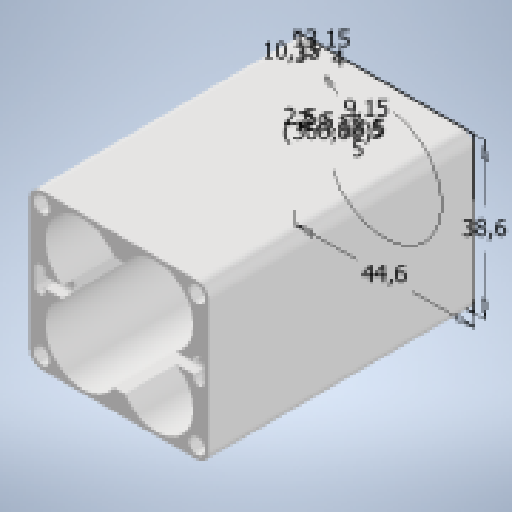
# Autodesk Inventor part: akkum
Saved by Autodesk Inventor 2025 (Build 290162000, 162)
## iProperties
Created: 2026-06-25
Part Number: akkum
Material: Типовые
Document SubType Name: Modeling
Designer: garin
Density: 1 g/cm^3
Appearance: По умолчанию
Author: garin
Autodesk Inventor part; units mm, degrees
ref_plane "YZ Plane" through (0, 0, 0) normal (1, 0, 0) x (0, 1, 0)
ref_plane "XZ Plane" through (0, 0, 0) normal (0, 1, 0) x (-1, 0, 0)
ref_plane "XY Plane" through (0, 0, 0) normal (0, 0, 1) x (1, 0, 0)
sketch "Эскиз1" plane through (0, 0, 0) normal (0, 0, 1) x (1, 0, 0)
  circle A0 centre (-9.15, 9.15) radius 9.25
  line L0 (0, 0) -> (-9.15, 0) construction
  line L1 (-9.15, 0) -> (-9.15, 9.15) construction
  line L2 (-9.15, 9.15) -> (0, 9.15) construction
  line L3 (0, 9.15) -> (0, 0) construction
  circle A1 centre (9.15, 9.15) radius 9.25
  circle A2 centre (-9.15, -9.15) radius 9.25
  circle A3 centre (9.15, -9.15) radius 9.25
  line L4 (0, 10.5065) -> (-0.6478, 10.5065) construction
  line L5 (-0.6478, 10.5065) -> (-0.6478, 5.5065) construction
  line L6 (-0.6478, 5.5065) -> (0, 5.5065) construction
  line L7 (0, 5.5065) -> (0, 10.5065) construction
  line L8 (-0.6478, 5.5065) -> (0.6478, 5.5065)
  line L9 (-0.6478, -5.5065) -> (0.6478, -5.5065)
  line L10 (-9.15, 0) -> (-4.15, 0) construction
  line L11 (-4.15, 0) -> (-4.15, 1.3678) construction
  line L12 (-4.15, 1.3678) -> (-9.15, 1.3678) construction
  line L13 (-9.15, 1.3678) -> (-9.15, 0) construction
  line L14 (-4.15, 1.3678) -> (-4.15, -1.3678)
  line L15 (4.15, 1.3678) -> (4.15, -1.3678)
  line L16 (-9.15, 9.15) -> (-22.3, 9.15) construction
  line L17 (-22.3, 9.15) -> (-22.3, 19.3) construction
  line L18 (-22.3, 19.3) -> (-9.15, 19.3) construction
  line L19 (-9.15, 19.3) -> (-9.15, 9.15) construction
  line L20 (-22.3, 19.3) -> (22.3, 19.3)
  line L21 (22.3, 19.3) -> (22.3, -19.3)
  line L22 (22.3, -19.3) -> (-22.3, -19.3)
  line L23 (-22.3, -19.3) -> (-22.3, 19.3)
  line L24 (-14.15, 1.3678) -> (-14.15, -1.3678)
  line L25 (14.15, 1.3678) -> (14.15, -1.3678)
  line L26 (-22.3, 19.3) -> (-19.3, 19.3) construction
  line L27 (-19.3, 19.3) -> (-19.3, 16.3) construction
  line L28 (-19.3, 16.3) -> (-22.3, 16.3) construction
  line L29 (-22.3, 16.3) -> (-22.3, 19.3) construction
  circle A4 centre (-19.3, 16.3) radius 2
  circle A5 centre (19.3, 16.3) radius 2
  circle A6 centre (-19.3, -16.3) radius 2
  circle A7 centre (19.3, -16.3) radius 2
  line L30 (-22.3, 0) -> (-19.8, 0) construction
  line L31 (-19.8, 0) -> (-19.8, 2) construction
  circle A8 centre (-19.8, 2) radius 1.25
  circle A9 centre (-19.8, -2) radius 1.25
  circle A10 centre (19.8, 2) radius 1.25
  circle A11 centre (19.8, -2) radius 1.25
  line L32 (-9.15, -9.15) -> (-22.3, -9.15) construction
  line L33 (-19.8, 2) -> (-21.05, 2) construction
  line L34 (-19.8, -2) -> (-21.05, -2) construction
  line L35 (-21.05, 2) -> (-21.05, -2)
  line L36 (-18.55, 2) -> (-18.55, -2)
  line L37 (21.05, 2) -> (21.05, -2)
  line L38 (18.55, 2) -> (18.55, -2)
  line L39 (14.15, 1.3678) -> (18.55, 1.3678)
  line L40 (14.15, -1.3678) -> (18.55, -1.3678)
  line L41 (-14.15, 1.3678) -> (-18.55, 1.3678)
  line L42 (-14.15, -1.3678) -> (-18.55, -1.3678)
  line L43 (-1.3678, -14.15) -> (1.3678, -14.15)
  line L44 (14.15, -1.3678) -> (14.15, 1.3678)
  line L45 (1.3678, 14.15) -> (-1.3678, 14.15)
  point P0 (14.15, 1.3678)
  point P1 (14.15, -1.3678)
  point P2 (-14.15, -1.3678)
  point P3 (-14.15, 1.3678)
  point P4 (4.15, -1.3678)
  point P5 (4.15, 1.3678)
  point P6 (-0.6478, -5.5065)
  point P7 (0.6478, -5.5065)
  point P8 (-18.55, -1.3678)
  point P9 (10.5065, 0)
  point P10 (0, -10.5065)
  point P11 (0, -7.7935)
  point P12 (-7.7935, 0)
  point P13 (-10.5065, 0)
  point P14 (7.7935, 0)
  point P15 (0, 7.7935)
  point P16 (0, 10.5065)
  dimension "d22" = 2.5
  dimension "d0" = 18.5
  dimension "d1" = 9.15
  dimension "d2" = 9.15
  dimension "d3" = 5
  dimension "d4" = 5
  dimension "d5" = 13.15
  dimension "d6" = 10.15
  dimension "d7" = 44.6
  dimension "d8" = 38.6
  dimension "d17" = 3
  dimension "d18" = 3
  dimension "d19" = 4
  dimension "d20" = 2.5
  dimension "d21" = 2
  dimension "d30" = 360
  constraints: 92 end point, 25 symmetric about line, 12 parallel, 11 perpendicular, 10 horizontal, 9 centre point, 4 point on circle, 4 point on line, 3 coincident, 2 vertical, 1 midpoint, 30 other
  measures "d0" diameter of A0
  measures "d1" distance of L1.end L2.end
  measures "d2" distance of L0.end L1.end
  measures "d3" distance of L5.end L4.end
  measures "d4" distance of L12.end L11.end
  measures "d5" distance of L17.end L18.end
  measures "d6" distance of L16.end L17.end
  measures "d7" distance of L21.end L22.end
  measures "d8" distance of L20.end L21.end
  measures "d17" distance of L27.end L28.end
  measures "d18" distance of L26.end L27.end
  measures "d19" diameter of A4
  measures "d20" distance of L30.start L30.end
  measures "d21" distance of L30.end L31.end
extrude "Выдавливание1" add sketch "Эскиз1" along normal blind 66 contours L24 L42 L36 L41 | L39 L38 L40 L25 | L20 L21 L22 L23
fillet "Сопряжение1" radius 3 4 edges at (22.3, 19.3, 33) (22.3, -19.3, 33) (-22.3, 19.3, 33) (-22.3, -19.3, 33)
extrude "Выдавливание2" cut sketch "Эскиз1" along normal blind 3 contours L24 L42 L36 L41 | L39 L38 L40 L25
extrude "Выдавливание3" cut sketch "Эскиз1" against normal blind 3 from surface at 66 contours L24 L42 L36 L41 | L39 L38 L40 L25
fillet "Сопряжение2" radius 1 8 edges at (-16.35, -1.3678, 3) (-16.35, 1.3678, 3) (16.35, 1.3678, 3) (16.35, -1.3678, 3) (16.35, -1.3678, 63) (16.35, 1.3678, 63) (-16.35, 1.3678, 63) (-16.35, -1.3678, 63)
